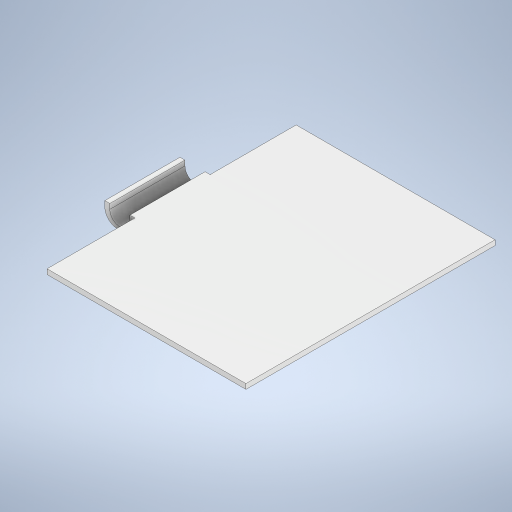
# Autodesk Inventor part: Battery Cover
Saved by Autodesk Inventor 2023 (Build 270158000, 158)
## iProperties
Created: 2022-11-17
Part Number: Battery Cover
Material: PC/ABS Plastic
Document SubType Name: Modeling
Designer: spfow
Density: 0.357273 g/cm^3
Appearance: Smooth - White
Author: spfow
Autodesk Inventor part; units mm, degrees
ref_plane "YZ Plane" through (0, 0, 0) normal (1, 0, 0) x (0, 1, 0)
ref_plane "XZ Plane" through (0, 0, 0) normal (0, 1, 0) x (-1, 0, 0)
ref_plane "XY Plane" through (0, 0, 0) normal (0, 0, 1) x (1, 0, 0)
sketch "Sketch1" plane through (0, 0, 0) normal (0, 1, 0) x (-1, 0, 0)
  line L0 (0, 0) -> (50.292, 0)
  line L1 (50.292, 0) -> (50.292, -62.992)
  line L2 (50.292, -62.992) -> (0, -62.992)
  line L3 (0, -62.992) -> (0, 0)
  line L4 (50.292, -22.225) -> (57.912, -22.225)
  line L5 (57.912, -22.225) -> (57.912, -41.2242)
  line L6 (57.912, -41.2242) -> (50.292, -41.2242)
  line L7 (50.292, -41.2242) -> (50.292, -22.225)
  dimension "d0" = 50.292
  dimension "d1" = 62.992
  dimension "d2" = 7.62
  dimension "d3" = 18.9992
  dimension "d4" = 22.225
  constraints: 16 end point, 4 parallel, 2 horizontal, 2 perpendicular, 1 point on line
  measures "d0" distance of L1.end L2.end
  measures "d1" distance of L0.end L1.end
  measures "d2" distance of L5.end L6.end
  measures "d3" distance of L4.end L5.end
  measures "d4" distance between parallel lines of L0 L4
extrude "Extrusion1" add sketch "Sketch1" against normal blind 1.27 contours L0 L1 L2 L3
extrude "Extrusion2" add sketch "Sketch1" against normal blind 4.572 contours L4 L5 L6 L1
sketch "Sketch2" plane through (-57.912, 0, -22.225) normal (0, 0, 1) x (1, 0, 0)
  line L0 (7.62, 0) -> (0, 0) projected
  line L1 (1.27, 0) -> (6.35, 0)
  line L2 (6.35, 0) -> (6.35, -1.27)
  line L3 (3.81, -3.81) -> (3.81, -3.81)
  line L4 (1.27, -1.27) -> (1.27, 0)
  line L5 (0, 0) -> (0, -4.572) projected
  arc A0 (1.27, -1.27) -> (3.81, -3.81) centre (3.81, -1.27) ccw
  arc A1 (3.81, -3.81) -> (6.35, -1.27) centre (3.81, -1.27) ccw
  point P0 (57.912, 0)
  point P1 (6.35, -3.81)
  point P2 (1.27, -3.81)
  point P3 (3.81, -3.81)
  point P4 (6.35, 0)
  dimension "d9" = 5.08
  dimension "d10" = 3.81
  dimension "d11" = 1.27
  dimension "d12" = 2.54
  dimension "d13" = 2.54
  constraints: 8 end point, 5 point on line, 4 point on circle, 4 tangent, 2 centre point, 2 parallel, 1 horizontal, 1 perpendicular
  measures "d9" distance of point (6.35, -3.81) point (1.27, -3.81)
  measures "d10" distance of point (1.27, -3.81) L1.start
  measures "d11" distance between parallel lines of L5 L4
  measures "d12" radius of A0
  measures "d13" radius of A1
extrude "Extrusion3" cut sketch "Sketch2" against normal through all
fillet "Fillet1" radius 3.175 2 edges at (-50.292, -4.572, -31.7246) (-57.912, -4.572, -31.7246)
body "Solid1"
